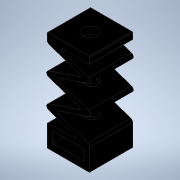
# Autodesk Inventor part: resorte5
Saved by Autodesk Inventor 2021.5 (Build 255421000, 421)
## iProperties
Created: 2024-11-28
Part Number: resorte5
Material: Genérico
Document SubType Name: Modeling
Designer: Joho_
Density: 1 g/cm^3
Appearance: Valor por defecto
Author: Joho_
## iProperties of the stored document _3DPrint.ipt
Created: 2024-11-28
Part Number: _3DPrint
Material: Genérico
Document SubType Name: Modeling
Designer: Joho_
Density: 1 g/cm^3
Appearance: Valor por defecto
Author: Joho_
Autodesk Inventor part; units mm, degrees
ref_plane "YZ Plane" through (0, 0, 0) normal (1, 0, 0) x (0, 1, 0)
ref_plane "XZ Plane" through (0, 0, 0) normal (0, 1, 0) x (-1, 0, 0)
ref_plane "XY Plane" through (0, 0, 0) normal (0, 0, 1) x (1, 0, 0)
sketch "Boceto1" plane through (0, 0, 0) normal (0, 0, 1) x (1, 0, 0)
  line L0 (-4.2, 2) -> (4.2, 2)
  line L1 (-4.4, 4.8) -> (-4.4, 2.2)
  line L2 (4.2, 5) -> (-4.2, 5)
  line L3 (4.4, 2.2) -> (4.4, 4.8)
  line L4 (6, 6.2) -> (6, 0.2)
  line L5 (-3, 6.2) -> (1.6383, 6.2)
  line L6 (-6, 0.2) -> (-6, 6)
  line L7 (-5.8, 0) -> (5.8, 0)
  line L8 (-5.8, 28.2) -> (5.8, 28.2)
  line L9 (6, 28) -> (6, 26.4)
  line L10 (5.8, 26.2) -> (-1.6383, 26.2)
  line L11 (-6, 26.1436) -> (-6, 28)
  line L12 (-3, 6.2) -> (-5.8, 6.2)
  line L13 (-5.1901, 10.47) -> (-5.0521, 10.516)
  line L14 (5.1901, 14.47) -> (5.0521, 14.516)
  line L15 (1.7647, 6.9795) -> (-5.622, 9.441)
  line L16 (-7.7794, 10.1599) -> (-7.7493, 10.2501)
  line L17 (7.7794, 6.2401) -> (7.4, 5.1016)
  line L18 (-5.622, 10.959) -> (2.9651, 13.8205)
  line L19 (7.7493, 14.2501) -> (7.7794, 14.1599)
  line L20 (-7.7493, 10.1499) -> (-7.7794, 10.2401)
  line L21 (2.9651, 14.5795) -> (-5.622, 17.441)
  line L22 (-7.7794, 18.1599) -> (-7.7493, 18.2501)
  line L23 (-2.9651, 17.8205) -> (5.622, 14.959)
  line L24 (7.7794, 14.2401) -> (7.7493, 14.1499)
  line L25 (-2.9651, 18.5795) -> (5.622, 21.441)
  line L26 (7.7794, 22.1599) -> (7.7493, 22.2501)
  line L27 (-7.7794, 18.2401) -> (-7.7493, 18.1499)
  line L28 (-1.7647, 25.4205) -> (5.622, 22.959)
  line L29 (7.7794, 22.2401) -> (7.7493, 22.1499)
  line L30 (6.0017, 22.8324) -> (6, 22.8319)
  line L31 (2.9651, 21.8205) -> (-5.622, 18.959)
  line L32 (6.0017, 21.5676) -> (6, 21.5681)
  line L33 (2.9651, 22.5795) -> (-5.4529, 25.3847)
  line L34 (-2.9651, 9.8205) -> (5.4529, 7.0153)
  line L35 (5.622, 13.441) -> (-2.9651, 10.5795)
  line L36 (-6, 9.5681) -> (-6.0017, 9.5676)
  line L37 (-6.0017, 10.8324) -> (-6, 10.8319)
  line L38 (-5.2246, 10.5735) -> (-5.0521, 10.516)
  line L39 (6, 6.2564) -> (6, 6.2)
  arc A0 (5.622, 21.441) -> (5.622, 22.959) centre (5.3691, 22.2) ccw
  arc A1 (-5.622, 18.959) -> (-5.622, 17.441) centre (-5.3691, 18.2) ccw
  arc A2 (5.622, 13.441) -> (5.622, 14.959) centre (5.3691, 14.2) ccw
  arc A3 (-5.622, 10.959) -> (-5.622, 9.441) centre (-5.3691, 10.2) ccw
  arc A4 (6, 6.2564) -> (5.4529, 7.0153) centre (5.2, 6.2564) ccw
  arc A5 (-6, 26.1436) -> (-5.4529, 25.3847) centre (-5.2, 26.1436) ccw
  arc A6 (-2.8711, 26.2) -> (-2.9343, 25.8103) centre (-2.8711, 26) ccw
  arc A7 (-3.5345, 18.3897) -> (-3.5345, 18.0103) centre (-3.4713, 18.2) ccw
  arc A8 (3.5345, 14.0103) -> (3.5345, 14.3897) centre (3.4713, 14.2) ccw
  arc A9 (-3.5345, 10.3897) -> (-3.5345, 10.0103) centre (-3.4713, 10.2) ccw
  arc A10 (2.8711, 6.2) -> (2.9343, 6.5897) centre (2.8711, 6.4) ccw
  arc A11 (-5.8, 6.2) -> (-6, 6) centre (-5.8, 6) ccw
  arc A12 (-6, 0.2) -> (-5.8, 0) centre (-5.8, 0.2) ccw
  arc A13 (5.8, 0) -> (6, 0.2) centre (5.8, 0.2) ccw
  arc A14 (-5.8, 28.2) -> (-6, 28) centre (-5.8, 28) ccw
  arc A15 (6, 28) -> (5.8, 28.2) centre (5.8, 28) ccw
  arc A16 (5.8, 26.2) -> (6, 26.4) centre (5.8, 26.4) ccw
  arc A17 (-4.2, 5) -> (-4.4, 4.8) centre (-4.2, 4.8) ccw
  arc A18 (-4.4, 2.2) -> (-4.2, 2) centre (-4.2, 2.2) ccw
  arc A19 (4.2, 2) -> (4.4, 2.2) centre (4.2, 2.2) ccw
  arc A20 (4.4, 4.8) -> (4.2, 5) centre (4.2, 4.8) ccw
  arc A21 (3.5345, 22.0103) -> (3.5345, 22.3897) centre (3.4713, 22.2) ccw
  arc A22 (2.9651, 21.8205) -> (2.9651, 22.5795) centre (2.8386, 22.2) ccw
  arc A23 (-2.9651, 18.5795) -> (-2.9651, 17.8205) centre (-2.8386, 18.2) ccw
  arc A24 (2.9651, 13.8205) -> (2.9651, 14.5795) centre (2.8386, 14.2) ccw
  arc A25 (-2.9651, 10.5795) -> (-2.9651, 9.8205) centre (-2.8386, 10.2) ccw
  arc A26 (1.6383, 6.2) -> (1.7647, 6.9795) centre (1.6383, 6.6) ccw
  arc A27 (-1.6383, 26.2) -> (-1.7647, 25.4205) centre (-1.6383, 25.8) ccw
  point P0 (0, 0)
  point P1 (0, 0)
  point P2 (6, 26.2)
  point P3 (6, 28.2)
  point P4 (6, 14.2)
  point P5 (6, 18.2)
  point P6 (6, 22.2)
  point P7 (-6, 10.2)
  point P8 (-6, 14.2)
  point P9 (-6, 18.2)
  point P10 (-6, 22.2)
  point P11 (0, 8.2)
  point P12 (0, 12.2)
  point P13 (0, 16.2)
  point P14 (0, 20.2)
  point P15 (0, 24.2)
  point P16 (4.1039, 22.2)
  dimension "d0" = 2
  dimension "d7" = 16
  dimension "d22" = 0.8
  dimension "d23" = 0.2
  dimension "d24" = 0.2
  dimension "d30" = 0.2
  dimension "d31" = 0.4
  constraints: 80 end point, 56 point on circle, 56 tangent, 46 point on line, 28 centre point, 23 equal radius, 16 parallel, 9 perpendicular, 1 horizontal, 1 vertical
  measures "d0" distance of point (6, 28.2) point (6, 26.2)
  measures "d7" distance of L17.end L16.start
  measures "d22" radius of A0
  measures "d23" radius of A6
  measures "d24" radius of A11
  measures "d30" radius of A21
  measures "d31" radius of A22
extrude "Extrusión1" add sketch "Boceto1" along normal mid plane 12
sketch "Boceto2" plane through (0, 0, 0) normal (0, 1, 0) x (-1, 0, 0)
  circle A0 centre (0, 0) radius 2
  dimension "d27" = 4
  constraints: 1 centre point, 1 coincident
  measures "d27" diameter of A0
extrude "Extrusión2" cut sketch "Boceto2" along normal blind 40
